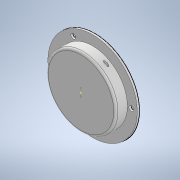
# Autodesk Inventor part: Return_Spool_Mount
Saved by Autodesk Inventor 2022 (Build 260153070, 153G)
## iProperties
Created: 2022-03-05
Part Number: Return_Spool_Mount
Material: Generic
Document SubType Name: Modeling
Designer: a laptop
Density: 1 g/cm^3
Appearance: Default
Author: a laptop
Autodesk Inventor part; units mm, degrees
ref_plane "YZ Plane" through (0, 0, 0) normal (1, 0, 0) x (0, 1, 0)
ref_plane "XZ Plane" through (0, 0, 0) normal (0, 1, 0) x (-1, 0, 0)
ref_plane "XY Plane" through (0, 0, 0) normal (0, 0, 1) x (1, 0, 0)
sketch "Sketch1" plane through (0, 0, 0) normal (0, 0, 1) x (1, 0, 0)
  circle A0 centre (0, 0) radius 55.075
  circle A1 centre (0, 0) radius 58.575
  circle A2 centre (0, 0) radius 75.075
  circle A3 centre (65.075, 0) radius 4
  circle A4 centre (-32.5375, 56.3566) radius 4
  circle A5 centre (-32.5375, -56.3566) radius 4
  line L0 (-32.5375, 56.3566) -> (-32.5375, -56.3566) construction
  line L1 (-32.5375, -56.3566) -> (65.075, 0) construction
  line L2 (65.075, 0) -> (-32.5375, 56.3566) construction
  line L3 (65.075, 0) -> (55.075, 0) construction
  line L4 (-32.5375, 56.3566) -> (-27.5375, 47.6963) construction
  line L5 (-27.5375, -47.6963) -> (-32.5375, -56.3566) construction
  dimension "d0" = 110.15
  dimension "d2" = 3.5
  dimension "d3" = 8
  dimension "d4" = 10
  dimension "d7" = 20
  constraints: 12 end point, 6 centre point, 4 equal length, 3 coincident, 3 line through centre, 3 point on circle, 2 equal radius, 1 horizontal
  measures "d0" diameter of A0
  measures "d2" radial gap between concentric circles of A0 A1
  measures "d3" diameter of A3
  measures "d4" distance of L0.start L4.end
  measures "d7" radial gap between concentric circles of A2 A0
extrude "Extrusion1" add sketch "Sketch1" along normal blind 3.5 contours A2
extrude "Extrusion2" add sketch "Sketch1" along normal blind 19.38 contours A1
sketch "Sketch2" plane through (0, 0, 19.38) normal (0, 0, 1) x (1, 0, 0)
  circle A0 centre (0, 0) radius 58.575 projected
  circle A1 centre (0, 6) radius 1.25
  circle A2 centre (0, -6) radius 1.25
  line L0 (0, -6) -> (0, 6)
  dimension "d13" = 2.5
  dimension "d14" = 12
  constraints: 2 centre point, 2 end point, 1 coincident, 1 equal radius, 1 midpoint, 1 vertical
  measures "d13" diameter of A1
  measures "d14" distance of L0.start L0.end
extrude "Extrusion3" add sketch "Sketch2" along normal blind 3.5
fillet "Fillet1" radius 3.5 2 edges at (-58.575, 0, 22.88) (-55.075, 0, 19.38)
sketch "Sketch3" plane through (0, 0, 0) normal (1, 0, 0) x (0, 1, 0)
  ellipse E0 centre (0, 10) end of major axis (-5, 10) minor radius 2
  line L0 (75.075, 0) -> (-75.075, 0) projected
  point P0 (0, 0)
  dimension "d15" = 5
  dimension "d17" = 2
  dimension "d16" = 10
  constraints: 1 vertical alignment, 2 other
  measures "d16" distance from line of L0 point (0, 10)
extrude "Extrusion4" cut sketch "Sketch3" against normal blind 76.75
pattern_circular "Circular Pattern1" count 3 over 360 about axis through (0, 0, -10) along (0, 0, 1) of "Extrusion4"
sketch "Sketch4" plane through (0, 0, 22.88) normal (0, 0, 1) x (1, 0, 0)
  point P0 (0, 0)
sketch "Sketch5" plane through (0, 0, 22.88) normal (0, 0, 1) x (1, 0, 0)
  circle A0 centre (0, 45) radius 6
  circle A1 centre (0, 45) radius 9 construction
  circle A2 centre (-7.7942, 49.5) radius 1.5
  circle A3 centre (7.7942, 49.5) radius 1.5
  circle A4 centre (0, 36) radius 1.5
  line L0 (-7.7942, 49.5) -> (7.7942, 49.5) construction
  line L1 (0, 36) -> (7.7942, 49.5) construction
  line L2 (-7.7942, 49.5) -> (0, 36) construction
  point P0 (0, 0)
  dimension "d23" = 12
  dimension "d24" = 18
  dimension "d25" = 3
  dimension "d26" = 45
  constraints: 6 end point, 5 centre point, 3 point on circle, 2 equal length, 2 equal radius, 1 coincident, 1 horizontal, 1 vertical alignment
  measures "d23" diameter of A0
  measures "d24" diameter of A1
  measures "d25" diameter of A4
  measures "d26" distance of point (0, 0) A0.centre
extrude "Extrusion5" cut sketch "Sketch5" against normal blind 10
body "Solid1"
